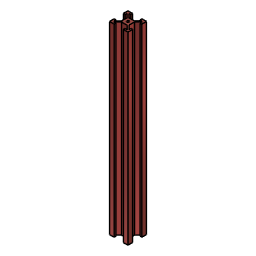
project cad chassis1 v11 (Autodesk Fusion 360 archive; units mm, degrees)
design "ROD Of Project"
Autodesk Fusion 360 part; units mm, degrees
sketch "Sketch1" plane through (0, 0, 0) normal (0, 0, 1) x (1, 0, 0)
  line L0 (10, 10) -> (-10, 10)
  line L1 (-10, 10) -> (-10, -10)
  line L2 (-10, -10) -> (10, -10)
  line L3 (10, -10) -> (10, 10)
  line L4 (4, 4) -> (-4, 4)
  line L5 (-4, 4) -> (-4, -4)
  line L6 (-4, -4) -> (4, -4)
  line L7 (4, -4) -> (4, 4)
  line L8 (-10, 10) -> (-5, 10)
  line L9 (-5, 10) -> (-5, 8.0163)
  line L10 (-10, 7) -> (-10, 10)
  line L11 (-10, 10) -> (-10, 5)
  line L12 (-10, 10) -> (-7, 10)
  line L13 (-8.1097, 5.0042) -> (-10, 5.0042)
  line L14 (-10, 5.0042) -> (-10, 10)
  line L15 (-5, 8.0163) -> (-8.1097, 8.0163)
  line L16 (-8.1097, 8.0163) -> (-8.1097, 5.0042)
  line L17 (8.0163, -5) -> (8.0163, -8.1097)
  line L18 (10, -5) -> (8.0163, -5)
  line L19 (8.0163, -8.1097) -> (5.0042, -8.1097)
  line L20 (5.0042, -8.1097) -> (5.0042, -10)
  line L21 (10, 10) -> (10, 5)
  line L22 (10, 10) -> (5, 10)
  line L23 (5, 10) -> (5, 7.9962)
  line L24 (5, 7.9962) -> (8.0438, 7.9962)
  line L25 (8.0438, 7.9962) -> (8.0438, 4.9845)
  line L26 (8.0438, 4.9845) -> (10, 5)
  line L27 (-7.9962, -8.0438) -> (-4.9845, -8.0438)
  line L28 (-4.9845, -8.0438) -> (-5, -10)
  line L29 (-7.9962, -5) -> (-7.9962, -8.0438)
  line L30 (-10, -5) -> (-7.9962, -5)
  line L31 (10, 10) -> (7.9962, 7.9962) construction
  line L32 (-2.926, 4) -> (-6.9956, 8.0163)
  line L33 (-4, 3.0393) -> (-8.1097, 7.0951)
  line L34 (2.9523, 4) -> (6.8961, 7.9962)
  line L35 (4, 3.0393) -> (8.0438, 7.1368)
  line L36 (4, -2.7637) -> (8.0163, -6.7273)
  line L37 (3.0653, -4) -> (7.2296, -8.1097)
  line L38 (-4, -2.9898) -> (-7.9962, -7.039)
  line L39 (-3.0014, -4) -> (-6.9922, -8.0438)
  circle A0 centre (0, 0) radius 1.1785
  dimension "d1" = 20
  constraint horizontal L0
  constraint perpendicular L0 L1
  constraint parallel L0 L2
  constraint parallel L1 L3
  constraint coincident A0.centre L31
  constraint coincident A0.centre origin
  constraint horizontal L4
  constraint perpendicular L4 L5
  constraint parallel L4 L6
  constraint parallel L5 L7
  constraint horizontal L8
  constraint vertical L9
  constraint vertical L10
  constraint horizontal L12
  constraint horizontal L13
  constraint vertical L14
  constraint perpendicular L9 L15
  constraint perpendicular L13 L16
  constraint symmetric L8.end L18.start L31
  constraint symmetric L13.end L20.end L31
  constraint symmetric L9.end L17.start L31
  constraint symmetric L15.end L17.end L31
  constraint symmetric L13.start L19.end L31
  constraint perpendicular L0 L21
  constraint perpendicular L3 L22
  constraint perpendicular L22 L23
  constraint perpendicular L23 L24
  constraint perpendicular L24 L25
  constraint coincident L24 L31.end
  constraint coincident L4 L32.start
  constraint coincident L15 L32.end
  constraint coincident L5 L33.start
  constraint coincident L16 L33.end
  constraint parallel L32 L33
  constraint coincident L4 L34.start
  constraint coincident L24 L34.end
  constraint perpendicular L32 L34
  constraint coincident L7 L35.start
  constraint coincident L25 L35.end
  constraint parallel L34 L35
  constraint coincident L7 L36.start
  constraint coincident L17 L36.end
  constraint perpendicular L35 L36
  constraint coincident L6 L37.start
  constraint coincident L19 L37.end
  constraint parallel L36 L37
  constraint coincident L5 L38.start
  constraint coincident L29 L38.end
  constraint perpendicular L37 L38
  constraint coincident L6 L39.start
  constraint coincident L27 L39.end
  constraint parallel L38 L39
  measures "d1" distance of L1.end L2.end
extrude "Extrude1" add sketch "Sketch1" along normal blind 400 contours L0 L3 L21 L22 L23 L24 L25 L26 | L0 L1 L8 L9 L10 L11 L12 L13 L14 L15 L16 | L2 L3 L17 L18 L19 L20 | L4 L7 L24 L25 L34 L35 | L4 L5 L15 L16 L32 L33 | L4 L5 L6 L7 | L6 L7 L17 L19 L36 L37 | L1 L2 L27 L28 L29 L30 | L5 L6 L27 L29 L38 L39 in component "Component"
sketch "Sketch2" plane through (0, 0, 0) normal (0, 0, 1) x (1, 0, 0)
extrude "Extrude2" cut 1 faces at (0.0507, -3.0584, 400) along direction (0, 0, -1) blind 200 in component "Component"
component "Component" placed x (1, 0, 0) y (0, 1, 0) z (0, 0, 1) at (0, 0, 0)

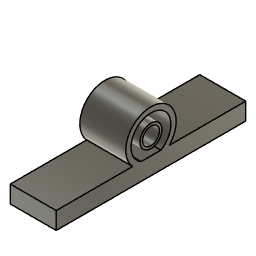
design "pillo"
Autodesk Fusion 360 part; units mm, degrees
sketch "Sketch1" plane through (0, 0, 0) normal (0, 0, 1) x (1, 0, 0)
  line L0 (8, 33) -> (-8, 33)
  line L1 (-8, 33) -> (-8, -33)
  line L2 (-8, -33) -> (8, -33)
  line L3 (8, -33) -> (8, 33)
  line L4 (8, 33) -> (-8, -33) construction
  line L5 (-8, 33) -> (8, -33) construction
  line L6 (-8, -33) -> (-8, -15)
  line L7 (-8, -15) -> (8, -15)
  line L8 (8, -15) -> (8, -33)
  line L9 (8, -33) -> (-8, -33)
  line L10 (-8, 33) -> (-8, 15)
  line L11 (-8, 15) -> (8, 15)
  line L12 (8, 15) -> (8, 33)
  line L13 (8, 33) -> (-8, 33)
  dimension "d1" = 16
  dimension "d2" = 66
  dimension "d3" = 18
  dimension "d4" = 18
  constraint horizontal L0
  constraint perpendicular L0 L1
  constraint parallel L0 L2
  constraint parallel L1 L3
  constraint coincident L4 origin
  constraint coincident L5 origin
  constraint perpendicular L2 L6
  constraint coincident L3 L7.end
  constraint perpendicular L3 L7
  constraint perpendicular L0 L10
  constraint coincident L3 L11.end
  constraint perpendicular L3 L11
  measures "d1" distance of L1.end L2.end
  measures "d2" distance of L0.end L1.end
  measures "d3" distance of L1.end L6.end
  measures "d4" distance of L0.end L10.end
extrude "Extrude1" add sketch "Sketch1" along normal blind 6 makes body 1
sketch "Sketch2" plane through (-8, 0, 0) normal (-1, 0, 0) x (0, -1, 0)
  line L0 (-33, 0) -> (33, 0)
  line L1 (33, 0) -> (33, 6)
  line L2 (33, 6) -> (-33, 6)
  line L3 (-33, 6) -> (-33, 0)
  circle A0 centre (0, 12.0275) radius 8.7885
  circle A1 centre (0, 12.0275) radius 8.0473
  circle A2 centre (0, 12.0275) radius 6.9543
  circle A3 centre (0, 12.0275) radius 3.7174
  circle A4 centre (0, 12.0275) radius 2.8253
  constraint concentric A0 A1
  constraint concentric A0 A2
  constraint concentric A1 A3
  constraint concentric A2 A4
extrude "Extrude2" add sketch "Sketch2" against normal blind 16 contours L2 A0 A1 | L2 A1 A2 picked at (-5.9628, 6.2834) picked at (-5.5281, 6.7137) bodies 1
sketch "Sketch3" plane through (-8, 0, 0) normal (-1, 0, 0) x (0, -1, 0)
  line L0 (-6.3958, 6) -> (-33, 6)
  line L1 (-33, 6) -> (-33, 0)
  line L2 (-33, 0) -> (33, 0)
  line L3 (33, 0) -> (33, 6)
  line L4 (33, 6) -> (6.3958, 6)
  arc A0 (6.3958, 6) -> (-6.3958, 6) centre (0, 12.0275) ccw
  arc A1 (3.4687, 6) -> (-3.4687, 6) centre (0, 12.0275) ccw
  line L5 (3.4687, 6) -> (-3.4687, 6)
  circle A2 centre (0, 12.0275) radius 3.833
  circle A3 centre (0, 12.0275) radius 2.9529
  constraint concentric A0 A2
  constraint concentric A2 A3
extrude "Extrude3" add sketch "Sketch3" against normal blind 16 separate body contours A2 makes body 2
sketch "Sketch4" plane through (0, 0, 0) normal (0, 1, 0) x (1, 0, 0)

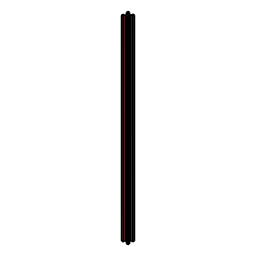
design "ROD Of Project"
Autodesk Fusion 360 part; units mm, degrees
sketch "Sketch1" plane through (0, 0, 0) normal (0, 0, 1) x (1, 0, 0)
  line L0 (10, 10) -> (-10, 10)
  line L1 (-10, 10) -> (-10, -10)
  line L2 (-10, -10) -> (10, -10)
  line L3 (10, -10) -> (10, 10)
  line L4 (4, 4) -> (-4, 4)
  line L5 (-4, 4) -> (-4, -4)
  line L6 (-4, -4) -> (4, -4)
  line L7 (4, -4) -> (4, 4)
  line L8 (-10, 10) -> (-5, 10)
  line L9 (-5, 10) -> (-5, 8.0163)
  line L10 (-10, 7) -> (-10, 10)
  line L11 (-10, 10) -> (-10, 5)
  line L12 (-10, 10) -> (-7, 10)
  line L13 (-8.1097, 5.0042) -> (-10, 5.0042)
  line L14 (-10, 5.0042) -> (-10, 10)
  line L15 (-5, 8.0163) -> (-8.1097, 8.0163)
  line L16 (-8.1097, 8.0163) -> (-8.1097, 5.0042)
  line L17 (8.0163, -5) -> (8.0163, -8.1097)
  line L18 (10, -5) -> (8.0163, -5)
  line L19 (8.0163, -8.1097) -> (5.0042, -8.1097)
  line L20 (5.0042, -8.1097) -> (5.0042, -10)
  line L21 (10, 10) -> (10, 5)
  line L22 (10, 10) -> (5, 10)
  line L23 (5, 10) -> (5, 7.9962)
  line L24 (5, 7.9962) -> (8.0438, 7.9962)
  line L25 (8.0438, 7.9962) -> (8.0438, 4.9845)
  line L26 (8.0438, 4.9845) -> (10, 5)
  line L27 (-7.9962, -8.0438) -> (-4.9845, -8.0438)
  line L28 (-4.9845, -8.0438) -> (-5, -10)
  line L29 (-7.9962, -5) -> (-7.9962, -8.0438)
  line L30 (-10, -5) -> (-7.9962, -5)
  line L31 (10, 10) -> (7.9962, 7.9962) construction
  line L32 (-2.926, 4) -> (-6.9956, 8.0163)
  line L33 (-4, 3.0393) -> (-8.1097, 7.0951)
  line L34 (2.9523, 4) -> (6.8961, 7.9962)
  line L35 (4, 3.0393) -> (8.0438, 7.1368)
  line L36 (4, -2.7637) -> (8.0163, -6.7273)
  line L37 (3.0653, -4) -> (7.2296, -8.1097)
  line L38 (-4, -2.9898) -> (-7.9962, -7.039)
  line L39 (-3.0014, -4) -> (-6.9922, -8.0438)
  circle A0 centre (0, 0) radius 1.1785
  dimension "d1" = 20
  constraint horizontal L0
  constraint perpendicular L0 L1
  constraint parallel L0 L2
  constraint parallel L1 L3
  constraint coincident A0.centre L31
  constraint coincident A0.centre origin
  constraint horizontal L4
  constraint perpendicular L4 L5
  constraint parallel L4 L6
  constraint parallel L5 L7
  constraint horizontal L8
  constraint vertical L9
  constraint vertical L10
  constraint horizontal L12
  constraint horizontal L13
  constraint vertical L14
  constraint perpendicular L9 L15
  constraint perpendicular L13 L16
  constraint symmetric L8.end L18.start L31
  constraint symmetric L13.end L20.end L31
  constraint symmetric L9.end L17.start L31
  constraint symmetric L15.end L17.end L31
  constraint symmetric L13.start L19.end L31
  constraint perpendicular L0 L21
  constraint perpendicular L3 L22
  constraint perpendicular L22 L23
  constraint perpendicular L23 L24
  constraint perpendicular L24 L25
  constraint coincident L24 L31.end
  constraint coincident L4 L32.start
  constraint coincident L15 L32.end
  constraint coincident L5 L33.start
  constraint coincident L16 L33.end
  constraint parallel L32 L33
  constraint coincident L4 L34.start
  constraint coincident L24 L34.end
  constraint perpendicular L32 L34
  constraint coincident L7 L35.start
  constraint coincident L25 L35.end
  constraint parallel L34 L35
  constraint coincident L7 L36.start
  constraint coincident L17 L36.end
  constraint perpendicular L35 L36
  constraint coincident L6 L37.start
  constraint coincident L19 L37.end
  constraint parallel L36 L37
  constraint coincident L5 L38.start
  constraint coincident L29 L38.end
  constraint perpendicular L37 L38
  constraint coincident L6 L39.start
  constraint coincident L27 L39.end
  constraint parallel L38 L39
  measures "d1" distance of L1.end L2.end
extrude "Extrude1" add sketch "Sketch1" along normal blind 600 contours L0 L3 L21 L22 L23 L24 L25 L26 | L0 L1 L8 L9 L10 L11 L12 L13 L14 L15 L16 | L2 L3 L17 L18 L19 L20 | L4 L7 L24 L25 L34 L35 | L4 L5 L15 L16 L32 L33 | L4 L5 L6 L7 | L6 L7 L17 L19 L36 L37 | L1 L2 L27 L28 L29 L30 | L5 L6 L27 L29 L38 L39 in component "Component"
component "Component" placed x (1, 0, 0) y (0, 1, 0) z (0, 0, 1) at (0, 0, 0)

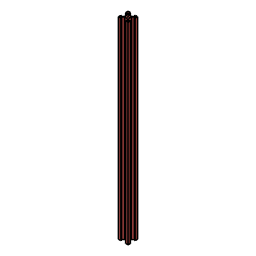
design "ROD Of Project"
Autodesk Fusion 360 part; units mm, degrees
sketch "Sketch1" plane through (0, 0, 0) normal (0, 0, 1) x (1, 0, 0)
  line L0 (10, 10) -> (-10, 10)
  line L1 (-10, 10) -> (-10, -10)
  line L2 (-10, -10) -> (10, -10)
  line L3 (10, -10) -> (10, 10)
  line L4 (4, 4) -> (-4, 4)
  line L5 (-4, 4) -> (-4, -4)
  line L6 (-4, -4) -> (4, -4)
  line L7 (4, -4) -> (4, 4)
  line L8 (-10, 10) -> (-5, 10)
  line L9 (-5, 10) -> (-5, 8.0163)
  line L10 (-10, 7) -> (-10, 10)
  line L11 (-10, 10) -> (-10, 5)
  line L12 (-10, 10) -> (-7, 10)
  line L13 (-8.1097, 5.0042) -> (-10, 5.0042)
  line L14 (-10, 5.0042) -> (-10, 10)
  line L15 (-5, 8.0163) -> (-8.1097, 8.0163)
  line L16 (-8.1097, 8.0163) -> (-8.1097, 5.0042)
  line L17 (8.0163, -5) -> (8.0163, -8.1097)
  line L18 (10, -5) -> (8.0163, -5)
  line L19 (8.0163, -8.1097) -> (5.0042, -8.1097)
  line L20 (5.0042, -8.1097) -> (5.0042, -10)
  line L21 (10, 10) -> (10, 5)
  line L22 (10, 10) -> (5, 10)
  line L23 (5, 10) -> (5, 7.9962)
  line L24 (5, 7.9962) -> (8.0438, 7.9962)
  line L25 (8.0438, 7.9962) -> (8.0438, 4.9845)
  line L26 (8.0438, 4.9845) -> (10, 5)
  line L27 (-7.9962, -8.0438) -> (-4.9845, -8.0438)
  line L28 (-4.9845, -8.0438) -> (-5, -10)
  line L29 (-7.9962, -5) -> (-7.9962, -8.0438)
  line L30 (-10, -5) -> (-7.9962, -5)
  line L31 (10, 10) -> (7.9962, 7.9962) construction
  line L32 (-2.926, 4) -> (-6.9956, 8.0163)
  line L33 (-4, 3.0393) -> (-8.1097, 7.0951)
  line L34 (2.9523, 4) -> (6.8961, 7.9962)
  line L35 (4, 3.0393) -> (8.0438, 7.1368)
  line L36 (4, -2.7637) -> (8.0163, -6.7273)
  line L37 (3.0653, -4) -> (7.2296, -8.1097)
  line L38 (-4, -2.9898) -> (-7.9962, -7.039)
  line L39 (-3.0014, -4) -> (-6.9922, -8.0438)
  circle A0 centre (0, 0) radius 1.1785
  dimension "d1" = 20
  constraint horizontal L0
  constraint perpendicular L0 L1
  constraint parallel L0 L2
  constraint parallel L1 L3
  constraint coincident A0.centre L31
  constraint coincident A0.centre origin
  constraint horizontal L4
  constraint perpendicular L4 L5
  constraint parallel L4 L6
  constraint parallel L5 L7
  constraint horizontal L8
  constraint vertical L9
  constraint vertical L10
  constraint horizontal L12
  constraint horizontal L13
  constraint vertical L14
  constraint perpendicular L9 L15
  constraint perpendicular L13 L16
  constraint symmetric L8.end L18.start L31
  constraint symmetric L13.end L20.end L31
  constraint symmetric L9.end L17.start L31
  constraint symmetric L15.end L17.end L31
  constraint symmetric L13.start L19.end L31
  constraint perpendicular L0 L21
  constraint perpendicular L3 L22
  constraint perpendicular L22 L23
  constraint perpendicular L23 L24
  constraint perpendicular L24 L25
  constraint coincident L24 L31.end
  constraint coincident L4 L32.start
  constraint coincident L15 L32.end
  constraint coincident L5 L33.start
  constraint coincident L16 L33.end
  constraint parallel L32 L33
  constraint coincident L4 L34.start
  constraint coincident L24 L34.end
  constraint perpendicular L32 L34
  constraint coincident L7 L35.start
  constraint coincident L25 L35.end
  constraint parallel L34 L35
  constraint coincident L7 L36.start
  constraint coincident L17 L36.end
  constraint perpendicular L35 L36
  constraint coincident L6 L37.start
  constraint coincident L19 L37.end
  constraint parallel L36 L37
  constraint coincident L5 L38.start
  constraint coincident L29 L38.end
  constraint perpendicular L37 L38
  constraint coincident L6 L39.start
  constraint coincident L27 L39.end
  constraint parallel L38 L39
  measures "d1" distance of L1.end L2.end
extrude "Extrude1" add sketch "Sketch1" along normal blind 400 contours L0 L3 L21 L22 L23 L24 L25 L26 | L0 L1 L8 L9 L10 L11 L12 L13 L14 L15 L16 | L2 L3 L17 L18 L19 L20 | L4 L7 L24 L25 L34 L35 | L4 L5 L15 L16 L32 L33 | L4 L5 L6 L7 | L6 L7 L17 L19 L36 L37 | L1 L2 L27 L28 L29 L30 | L5 L6 L27 L29 L38 L39 in component "Component"
component "Component" placed x (1, 0, 0) y (0, 1, 0) z (0, 0, 1) at (0, 0, 0)

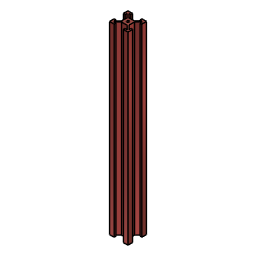
design "ROD Of Project"
Autodesk Fusion 360 part; units mm, degrees
sketch "Sketch1" plane through (0, 0, 0) normal (0, 0, 1) x (1, 0, 0)
  line L0 (10, 10) -> (-10, 10)
  line L1 (-10, 10) -> (-10, -10)
  line L2 (-10, -10) -> (10, -10)
  line L3 (10, -10) -> (10, 10)
  line L4 (4, 4) -> (-4, 4)
  line L5 (-4, 4) -> (-4, -4)
  line L6 (-4, -4) -> (4, -4)
  line L7 (4, -4) -> (4, 4)
  line L8 (-10, 10) -> (-5, 10)
  line L9 (-5, 10) -> (-5, 8.0163)
  line L10 (-10, 7) -> (-10, 10)
  line L11 (-10, 10) -> (-10, 5)
  line L12 (-10, 10) -> (-7, 10)
  line L13 (-8.1097, 5.0042) -> (-10, 5.0042)
  line L14 (-10, 5.0042) -> (-10, 10)
  line L15 (-5, 8.0163) -> (-8.1097, 8.0163)
  line L16 (-8.1097, 8.0163) -> (-8.1097, 5.0042)
  line L17 (8.0163, -5) -> (8.0163, -8.1097)
  line L18 (10, -5) -> (8.0163, -5)
  line L19 (8.0163, -8.1097) -> (5.0042, -8.1097)
  line L20 (5.0042, -8.1097) -> (5.0042, -10)
  line L21 (10, 10) -> (10, 5)
  line L22 (10, 10) -> (5, 10)
  line L23 (5, 10) -> (5, 7.9962)
  line L24 (5, 7.9962) -> (8.0438, 7.9962)
  line L25 (8.0438, 7.9962) -> (8.0438, 4.9845)
  line L26 (8.0438, 4.9845) -> (10, 5)
  line L27 (-7.9962, -8.0438) -> (-4.9845, -8.0438)
  line L28 (-4.9845, -8.0438) -> (-5, -10)
  line L29 (-7.9962, -5) -> (-7.9962, -8.0438)
  line L30 (-10, -5) -> (-7.9962, -5)
  line L31 (10, 10) -> (7.9962, 7.9962) construction
  line L32 (-2.926, 4) -> (-6.9956, 8.0163)
  line L33 (-4, 3.0393) -> (-8.1097, 7.0951)
  line L34 (2.9523, 4) -> (6.8961, 7.9962)
  line L35 (4, 3.0393) -> (8.0438, 7.1368)
  line L36 (4, -2.7637) -> (8.0163, -6.7273)
  line L37 (3.0653, -4) -> (7.2296, -8.1097)
  line L38 (-4, -2.9898) -> (-7.9962, -7.039)
  line L39 (-3.0014, -4) -> (-6.9922, -8.0438)
  circle A0 centre (0, 0) radius 1.1785
  dimension "d1" = 20
  constraint horizontal L0
  constraint perpendicular L0 L1
  constraint parallel L0 L2
  constraint parallel L1 L3
  constraint coincident A0.centre L31
  constraint coincident A0.centre origin
  constraint horizontal L4
  constraint perpendicular L4 L5
  constraint parallel L4 L6
  constraint parallel L5 L7
  constraint horizontal L8
  constraint vertical L9
  constraint vertical L10
  constraint horizontal L12
  constraint horizontal L13
  constraint vertical L14
  constraint perpendicular L9 L15
  constraint perpendicular L13 L16
  constraint symmetric L8.end L18.start L31
  constraint symmetric L13.end L20.end L31
  constraint symmetric L9.end L17.start L31
  constraint symmetric L15.end L17.end L31
  constraint symmetric L13.start L19.end L31
  constraint perpendicular L0 L21
  constraint perpendicular L3 L22
  constraint perpendicular L22 L23
  constraint perpendicular L23 L24
  constraint perpendicular L24 L25
  constraint coincident L24 L31.end
  constraint coincident L4 L32.start
  constraint coincident L15 L32.end
  constraint coincident L5 L33.start
  constraint coincident L16 L33.end
  constraint parallel L32 L33
  constraint coincident L4 L34.start
  constraint coincident L24 L34.end
  constraint perpendicular L32 L34
  constraint coincident L7 L35.start
  constraint coincident L25 L35.end
  constraint parallel L34 L35
  constraint coincident L7 L36.start
  constraint coincident L17 L36.end
  constraint perpendicular L35 L36
  constraint coincident L6 L37.start
  constraint coincident L19 L37.end
  constraint parallel L36 L37
  constraint coincident L5 L38.start
  constraint coincident L29 L38.end
  constraint perpendicular L37 L38
  constraint coincident L6 L39.start
  constraint coincident L27 L39.end
  constraint parallel L38 L39
  measures "d1" distance of L1.end L2.end
extrude "Extrude1" add sketch "Sketch1" along normal blind 400 contours L0 L3 L21 L22 L23 L24 L25 L26 | L0 L1 L8 L9 L10 L11 L12 L13 L14 L15 L16 | L2 L3 L17 L18 L19 L20 | L4 L7 L24 L25 L34 L35 | L4 L5 L15 L16 L32 L33 | L4 L5 L6 L7 | L6 L7 L17 L19 L36 L37 | L1 L2 L27 L28 L29 L30 | L5 L6 L27 L29 L38 L39 in component "Component"
sketch "Sketch2" plane through (0, 0, 0) normal (0, 0, 1) x (1, 0, 0)
extrude "Extrude2" cut 1 faces at (0.0507, -3.0584, 400) along direction (0, 0, -1) blind 200 in component "Component"
component "Component" placed x (1, 0, 0) y (0, 1, 0) z (0, 0, 1) at (0, 0, 0)

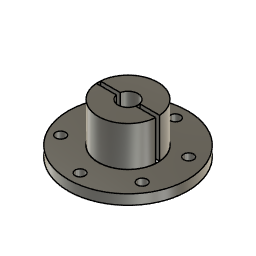
design "project capling"
Autodesk Fusion 360 part; units mm, degrees
sketch "Sketch1" plane through (0, 0, 0) normal (0, 0, 1) x (1, 0, 0)
  circle A0 centre (0, 0) radius 30
  circle A1 centre (0, 0) radius 15
  circle A2 centre (0, 23.8555) radius 2.5
  circle A3 centre (0, -24.1295) radius 2.5
  circle A4 centre (20.3573, 10.1786) radius 2.5
  circle A5 centre (-20.6734, 10.8741) radius 2.5
  circle A6 centre (19.6619, -12.5389) radius 2.5074
  circle A7 centre (-21.3688, -12.5389) radius 2.5
  dimension "d1" = 60
  dimension "d2" = 30
  dimension "d3" = 5
  dimension "d4" = 5
  dimension "d5" = 5
  dimension "d6" = 5
  dimension "d7" = 5
  constraint coincident A0.centre A1.centre
  constraint concentric A0 A1
  measures "d1" diameter of A0
  measures "d2" diameter of A1
  measures "d3" diameter of A2
  measures "d4" diameter of A3
  measures "d5" diameter of A4
  measures "d6" diameter of A5
  measures "d7" diameter of A7
extrude "Extrude1" add sketch "Sketch1" along normal blind 5 makes body 1
sketch "Sketch2" plane through (0, 0, 5) normal (0, 0, 1) x (-1, 0, 0)
  circle A0 centre (0, 0) radius 15
  circle A1 centre (21.3688, 12.5389) radius 2.5
  circle A2 centre (20.6734, -10.8741) radius 2.5
  circle A3 centre (0, -23.8555) radius 2.5
  circle A4 centre (-20.3573, -10.1786) radius 2.5
  circle A5 centre (-19.6619, 12.5389) radius 2.5074
  circle A6 centre (0, 24.1295) radius 2.5
  circle A7 centre (0, 0) radius 30
  circle A8 centre (0, 0) radius 14.9388
  constraint coincident A0.centre A7.centre
extrude "Extrude2" add sketch "Sketch2" along normal blind 20 separate body contours A8 makes body 2
sketch "Sketch3" plane through (0, 0, 25) normal (0, 0, 1) x (-1, 0, 0)
  circle A0 centre (0, 0) radius 14.9388
  circle A1 centre (0, 0) radius 5
  dimension "d12" = 10
  constraint coincident A0.centre A1.centre
  measures "d12" diameter of A1
extrude "Extrude3" cut sketch "Sketch3" against normal blind 50 contours A1 bodies 2
sketch "Sketch4" plane through (0, 0, 25) normal (0, 0, 1) x (-1, 0, 0)
  circle A0 centre (0, 0) radius 5
  circle A1 centre (0, 0) radius 14.9388
  line L0 (-5.0555, 1) -> (-15.0555, 1)
  line L1 (-15.0555, 1) -> (-15.0555, -1)
  line L2 (-15.0555, -1) -> (-5.0555, -1)
  line L3 (-5.0555, -1) -> (-5.0555, 1)
  line L4 (-5.0555, 1) -> (-15.0555, -1) construction
  line L5 (-15.0555, 1) -> (-5.0555, -1) construction
  line L6 (14.8415, 1) -> (4.8415, 1)
  line L7 (4.8415, 1) -> (4.8415, -1)
  line L8 (4.8415, -1) -> (14.8415, -1)
  line L9 (14.8415, -1) -> (14.8415, 1)
  line L10 (14.8415, 1) -> (4.8415, -1) construction
  line L11 (4.8415, 1) -> (14.8415, -1) construction
  point P0 (-10.0555, 0)
  point P1 (9.8415, 0)
  dimension "d15" = 10
  dimension "d16" = 2
  dimension "d17" = 10
  dimension "d18" = 2
  constraint horizontal L0
  constraint perpendicular L0 L1
  constraint parallel L0 L2
  constraint parallel L1 L3
  constraint coincident L4 P0
  constraint coincident L5 P0
  constraint horizontal L6
  constraint perpendicular L6 L7
  constraint parallel L6 L8
  constraint parallel L7 L9
  constraint coincident L10 P1
  constraint coincident L11 P1
  measures "d15" distance of L1.end L2.end
  measures "d16" distance of L0.end L1.end
  measures "d17" distance of L7.end L8.end
  measures "d18" distance of L6.end L7.end
extrude "Extrude4" cut sketch "Sketch4" against normal blind 20 contours A0 L6 L8 L9 | A1 L0 L2 L3 picked at (-8.3487, -0.1112) bodies 2
